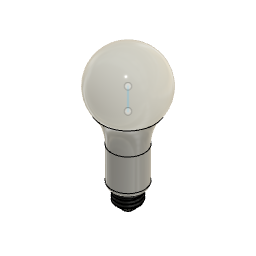
gyakorlati 6 villanykorte (Autodesk Fusion 360 design; units mm, degrees)
Autodesk Fusion 360 part; units mm, degrees
cylinder "CylinderPrimitive1" add diameter 30 height 55 placed x (1, 0, 0) y (0, 1, 0) z (0, 0, 1) at (0, 0, 0) makes body 1
sketch "Sketch2" plane through (0, 0, 0) normal (0, 1, 0) x (1, 0, 0)
  line L0 (0, -60) -> (0, -80)
  dimension "d3" = 20
  constraint vertical L0
  measures "d3" distance of L0.start L0.end
sphere "SpherePrimitive1" add diameter 61 placed x (1, 0, 0) y (0, 0, -1) z (0, 1, 0) at (0, 0, 80) bodies 1
fillet "Fillet1" radius 45 1 edges at (-13.9849, 5.4242, 53.4435) on bodies 1
fillet "Fillet2" radius 5 1 edges at (-13.9849, 5.4242, 0) on bodies 1
cylinder "CylinderPrimitive2" add diameter 22 height 15 placed x (0, 1, 0) y (1, 0, 0) z (0, 0, -1) at (0, 0, 0) separate body makes body 2
thread "Thread1" "ANSI Metric M Profile 22.0 M22x3 6g" major diameter 21.7645 minor diameter 18.3374 pitch 3 angle 60 modelled right hand crest width 0.4298 on face at (-1.0952, 10.9453, -5) from (0, 0, -2) to (0, 0, -12) crest through (0, 10.8823, 0.75) on bodies 2
chamfer "Chamfer1" distance 5 angle 45 1 edges at (-3.9352, -10.1458, -15) on bodies 2
cylinder "CylinderPrimitive3" add diameter 11.765 height 2 placed x (0, 1, 0) y (1, 0, 0) z (0, 0, -1) at (0, 0, -15) bodies 2
chamfer "Chamfer2" distance 2 angle 45 1 edges at (-2.1272, -5.4844, -17) on bodies 2
